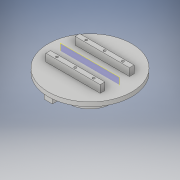
# Autodesk Inventor part: turntable
Saved by Autodesk Inventor 2018 (Build 220112000, 112)
## iProperties
Created: 2020-02-28
Part Number: turntable
Material: Generisch
Document SubType Name: Modeling
Designer: Tanja
Density: 1 g/cm^3
Appearance: Vorgabe
Author: Tanja
Autodesk Inventor part; units mm, degrees
ref_plane "YZ Plane" through (0, 0, 0) normal (1, 0, 0) x (0, 1, 0)
ref_plane "XZ Plane" through (0, 0, 0) normal (0, 1, 0) x (-1, 0, 0)
ref_plane "XY Plane" through (0, 0, 0) normal (0, 0, 1) x (1, 0, 0)
sketch "Skizze1" plane through (0, 0, 0) normal (0, 0, 1) x (1, 0, 0)
  circle A0 centre (0, 0) radius 50
  dimension "d0" = 100
  constraints: 1 centre point, 1 coincident
  measures "d0" diameter of A0
extrude "Extrusion1" add sketch "Skizze1" along normal blind 5
sketch "Skizze2" plane through (0, 0, 0) normal (0, 0, -1) x (-1, 0, 0)
  circle A0 centre (0, 0) radius 6
  circle A1 centre (0, 0) radius 8
  dimension "d3" = 12
  dimension "d4" = 16
  constraints: 2 centre point, 2 coincident
  measures "d3" diameter of A0
  measures "d4" diameter of A1
extrude "Extrusion2" add sketch "Skizze2" along normal blind 20
sketch "Skizze3" plane through (0, 0, 0) normal (0, 0, -1) x (-1, 0, 0)
  circle A0 centre (0, 0) radius 50 construction
  line L0 (50, 0) -> (40, 0) construction
  line L1 (40, 0) -> (40, 5) construction
  line L2 (40, 5) -> (50, 5) construction
  line L3 (40, 5) -> (50, 5) construction
  line L4 (50, 5) -> (50, 0) construction
  line L5 (50, 0) -> (50, -5) construction
  line L6 (40, 5) -> (50, 5)
  line L7 (50, 5) -> (50, -5)
  line L8 (50, -5) -> (40, -5)
  line L9 (40, -5) -> (40, 5)
  dimension "d7" = 10
  dimension "d8" = 5
  dimension "d10" = 10
  dimension "d11" = 0
  dimension "d12" = 5
  constraints: 20 end point, 4 horizontal, 2 parallel, 2 perpendicular, 2 vertical, 1 collinear, 1 horizontal alignment, 1 other
  measures "d7" distance of L0.start L0.end
  measures "d8" distance of L0.end L1.end
  measures "d10" distance of L1.end L2.end
  measures "d11" distance between parallel lines of L2 L3
  measures "d12" distance of L0.start L5.end
extrude "Extrusion3" add sketch "Skizze3" along normal blind 50
sketch "Skizze4" plane through (0, 0, 5) normal (0, 0, 1) x (1, 0, 0)
  line L0 (-40, 5) -> (-49.7494, 5) construction
  circle A0 centre (0, 0) radius 6 construction
  line L1 (0, 0) -> (32.55, 0) construction
  line L2 (32.55, 0) -> (32.55, -20.3)
  line L3 (0, 0) -> (-32.55, 0) construction
  line L4 (-32.55, 0) -> (-32.55, -20.3) construction
  line L5 (-32.55, 0) -> (-32.55, -20.3) construction
  line L6 (32.55, -20.3) -> (32.55, -14.7) construction
  line L7 (-32.55, -20.3) -> (-32.55, -14.7) construction
  line L8 (-32.55, -20.3) -> (32.55, -20.3)
  line L9 (32.55, -20.3) -> (32.55, -14.7)
  line L10 (32.55, -14.7) -> (-32.55, -14.7)
  line L11 (-32.55, -14.7) -> (-32.55, -20.3)
  dimension "d23" = 32.55
  dimension "d24" = 20.3
  dimension "d25" = 32.55
  dimension "d26" = 20.3
  dimension "d27" = 5.6
  dimension "d28" = 5.6
  constraints: 22 end point, 3 equal length, 3 horizontal, 3 perpendicular, 2 point on line
  measures "d23" distance of L1.start L1.end
  measures "d24" distance of L1.end L2.end
  measures "d25" distance of L1.start L3.end
  measures "d26" distance of L3.end L4.end
  measures "d27" distance of L2.end L6.end
  measures "d28" distance of L4.end L7.end
extrude "Extrusion4" add sketch "Skizze4" along normal blind 9
ref_plane "Arbeitsebene1" through (-32.55, 0, 5) normal (0, 1, 0) x (1, 0, 0)
mirror "Spiegeln1" about plane through (-32.55, 0, 5) normal (0, 1, 0) of "Extrusion4"
sketch "Skizze9" plane through (-32.55, 20.3, 14) normal (0, 0, 1) x (1, 0, 0)
  circle A0 centre (32.5, -2.8) radius 1.35 projected
  circle A1 centre (54.5, -2.8) radius 1.35 projected
  circle A2 centre (10.5, -2.8) radius 1.35 projected
  circle A3 centre (54.5, -2.8) radius 1.4
  circle A4 centre (32.5, -2.8) radius 1.4
  circle A5 centre (10.5, -2.8) radius 1.4
  point P0 (32.55, -20.3)
  dimension "d40" = 2.8
  dimension "d41" = 2.8
  dimension "d42" = 2.8
  constraints: 3 centre point, 3 coincident
  measures "d40" diameter of A3
  measures "d41" diameter of A4
  measures "d42" diameter of A5
extrude "Extrusion7" cut sketch "Skizze9" against normal through all contours A0 | A1 | A2
mirror "Spiegeln3" about plane through (-32.55, 0, 5) normal (0, 1, 0) of "Extrusion7"
sketch "Skizze11" plane through (0, 0, -20) normal (0, 0, -1) x (-1, 0, 0)
  circle A0 centre (0, 0) radius 8 projected
  circle A1 centre (0, 0) radius 8
  circle A2 centre (0, 0) radius 25
  dimension "d53" = 16
  dimension "d54" = 50
  constraints: 2 centre point, 2 coincident
  measures "d53" diameter of A1
  measures "d54" diameter of A2
extrude "Extrusion9" add sketch "Skizze11" against normal blind 5
